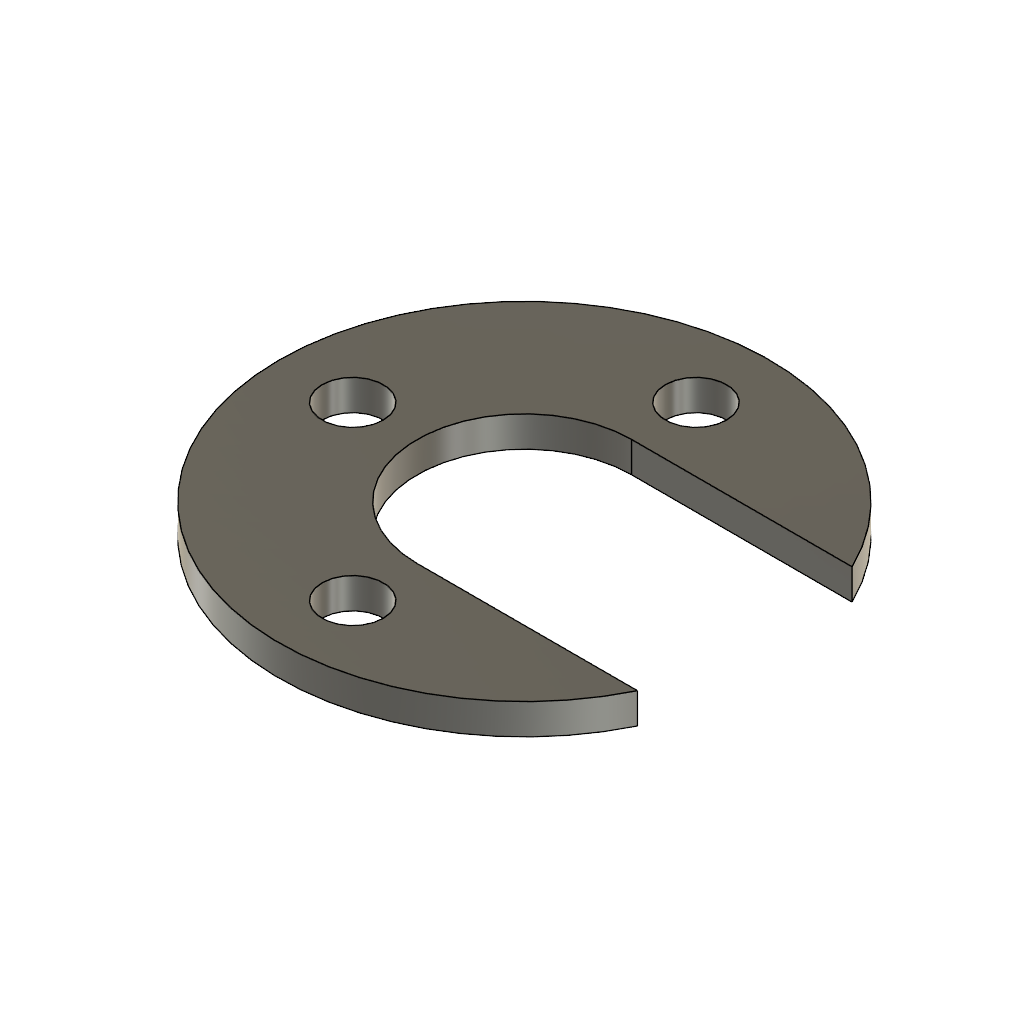
exercise 1 (Autodesk Fusion 360 design; units mm, degrees)
part number: 2026-10-01-22-02-10-759
Autodesk Fusion 360 part; units mm, degrees
sketch "Sketch1" plane through (0, 0, 0) normal (0, 0, 1) x (1, 0, 0)
  circle A0 centre (0, 28) radius 5
  circle A1 centre (-28, 0) radius 5
  circle A2 centre (0, -28) radius 5
  line L0 (0, 17.5) -> (35.9687, 17.5)
  line L1 (0, -17.5) -> (35.9687, -17.5)
  arc A3 (35.9687, 17.5) -> (35.9687, -17.5) centre (0, 0) ccw
  arc A4 (0, 17.5) -> (0, -17.5) centre (0, 0) ccw
  dimension "d1" = 80
  dimension "d2" = 35
  dimension "d3" = 28
  dimension "d4" = 10
  dimension "d6" = 180
  constraint coincident A3.centre A4.centre
  constraint tangent L0 A4
  constraint horizontal L0
  constraint tangent L1 A4
  constraint horizontal L1
  measures "d1" diameter of A3
  measures "d2" diameter of A4
  measures "d3" distance of A3.centre A0.centre
  measures "d4" diameter of A0
extrude "Extrude1" add sketch "Sketch1" along normal blind 5
